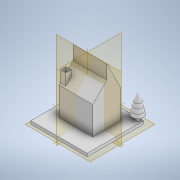
# Autodesk Inventor part: House_Assembly_Depth_Tracking
Saved by Autodesk Inventor 2022.4 (Build 264492010, 492A)
## iProperties
Created: 2025-04-13
Part Number: House_Assembly_Depth_Tracking
Material: Generic
Document SubType Name: Modeling
Designer: jan-m
Density: 1 g/cm^3
Appearance: Default
Author: jan-m
Autodesk Inventor part; units mm, degrees
sketch "Sketch1" plane through (0, 0, 0) normal (1, 0, 0) x (0, 1, 0)
  line L0 (11, 100) -> (0, 100)
  line L1 (0, 100) -> (0, -100)
  line L2 (0, -100) -> (11, -100)
  line L3 (11, -100) -> (11, 100)
  line L4 (-2.2, 0) -> (13.2, 0) projected
  line L5 (0, 140) -> (0, -140) projected
  point P0 (0, 0)
  point P1 (11, 0)
  dimension "d0" = 200
  dimension "d1" = 11
  dimension "d2" = 0
  constraints: 8 end point, 2 parallel, 1 horizontal, 1 midpoint, 1 perpendicular, 1 point on line
  measures "d0" distance of L2.end L0.start
  measures "d1" distance of L1.end L2.end
  measures "d2" distance between parallel lines of L5 L1
extrude "Extrusion1" add sketch "Sketch1" along normal mid plane 200
sketch "Sketch2" plane through (0, 0, 0) normal (1, 0, 0) x (0, 1, 0)
  line L0 (111, 40) -> (11, 40)
  line L1 (11, 40) -> (11, -60)
  line L2 (11, -60) -> (111, -60)
  line L3 (111, -60) -> (111, 40)
  line L4 (-32.1032, 0) -> (192.619, 0) projected
  line L5 (11, -100) -> (11, 100) projected
  line L6 (111, 40) -> (161, 40)
  line L7 (161, 40) -> (161, -10)
  line L8 (161, -10) -> (111, -10)
  line L9 (111, -10) -> (111, 40)
  line L10 (111, -60) -> (211, -60)
  line L11 (211, -60) -> (211, -10)
  line L12 (211, -10) -> (111, -10)
  line L13 (111, -10) -> (111, -60)
  line L14 (111, 40) -> (161, -10)
  line L15 (111, -60) -> (211, -10)
  point P0 (0, 0)
  dimension "d5" = 100
  dimension "d6" = 40
  dimension "d7" = 100
  dimension "d8" = 0
  dimension "d9" = 50
  dimension "d10" = 50
  dimension "d11" = 100
  dimension "d12" = 50
  constraints: 28 end point, 6 parallel, 3 horizontal, 3 perpendicular
  measures "d5" distance of L1.end L2.end
  measures "d6" distance between parallel lines of L4 L0
  measures "d7" distance of L2.end L0.start
  measures "d8" distance between parallel lines of L5 L1
  measures "d9" distance of L7.end L8.end
  measures "d10" distance of L6.end L7.end
  measures "d11" distance of L12.end L11.end
  measures "d12" distance of L11.end L10.end
extrude "Extrusion2" add sketch "Sketch2" along normal mid plane 120 contours L3 L4 L1 L0 | L14 L4 L3 | L4 L14 L8 L3 | L3 L2 L1 L4 | L8 L12 L15 L3
sketch "Sketch3" plane through (-60, 0, 0) normal (-1, 0, 0) x (0, 0, 1)
  line L0 (15.607, 155.393) -> (35.607, 155.393)
  line L1 (35.607, 155.393) -> (35.607, 135.393)
  line L2 (35.607, 135.393) -> (15.607, 135.393)
  line L3 (15.607, 135.393) -> (15.607, 155.393)
  line L4 (40, 111) -> (-10, 161) projected
  line L5 (35.607, 135.393) -> (35.607, 115.393)
  line L6 (-10, 161) -> (40, 111) projected
  line L7 (15.607, 135.393) -> (35.607, 115.393)
  point P0 (0, 0)
  dimension "d15" = 20
  dimension "d16" = 20
  dimension "d17" = 4.393
  constraints: 12 end point, 2 parallel, 2 point on line, 1 horizontal, 1 perpendicular, 1 vertical
  measures "d15" distance of L1.end L2.end
  measures "d16" distance of L0.end L1.end
  measures "d17" distance from line of L4.start L5
extrude "Extrusion3" add sketch "Sketch3" against normal blind 20
sketch "Sketch4" plane through (-60, 155.393, 35.607) normal (0, 1, 0) x (1, 0, 0)
  line L0 (20, 20) -> (20, 0) projected
  line L1 (0, 20) -> (20, 20) projected
  line L2 (0, 0) -> (0, 20) projected
  line L3 (0, 0) -> (20, 0) projected
  line L4 (18, 2) -> (18, 18)
  line L5 (18, 18) -> (2, 18)
  line L6 (2, 18) -> (2, 2)
  line L7 (2, 2) -> (18, 2)
  point P0 (60, 35.607)
  dimension "d20" = 2
  constraints: 8 end point, 3 other
  measures "d20" distance between parallel lines of L0 L4
extrude "Extrusion4" cut sketch "Sketch4" against normal blind 20 contours L7 L6 L5 L4
sketch "Sketch5" plane through (-100, 11, 100) normal (0, 1, 0) x (1, 0, 0)
  line L0 (200, 200) -> (200, 0) projected
  line L1 (0, 200) -> (200, 200) projected
  point P0 (100, 100)
  point P1 (190, 190)
  dimension "d23" = 10
  dimension "d24" = 10
  measures "d23" distance from line of L0 point (190, 190)
  measures "d24" distance from line of L1 point (190, 190)
ref_plane "Work Plane1" through (90, 11, -90) normal (1, 0, 0) x (0, 1, 0)
sketch "Sketch7" plane through (90, 11, -90) normal (1, 0, 0) x (0, 1, 0)
  line L0 (0, -10) -> (0, 190) projected
  line L1 (0, 0) -> (20, 0)
  line L2 (20, 0) -> (20, 5)
  line L3 (20, 5) -> (0, 5)
  line L4 (0, 5) -> (0, 0)
  line L5 (20, 0) -> (20, 20)
  line L6 (90, 0) -> (60.481, 11.7284)
  line L7 (60.481, 11.7284) -> (60.481, 5)
  line L8 (60.481, 9.4368) -> (46.541, 14.9754)
  line L9 (46.541, 14.9754) -> (46.541, 5)
  line L10 (46.541, 12.5046) -> (32.601, 18.0432)
  line L11 (32.601, 18.0432) -> (32.601, 5)
  line L12 (32.601, 15.2739) -> (20, 20)
  line L13 (90, 0) -> (20, 0)
  point P0 (-11, 90)
  dimension "d25" = 20
  dimension "d26" = 5
  dimension "d27" = 20
  dimension "d28" = 15
  dimension "d29" = 15
  constraints: 26 end point, 4 parallel, 3 point on line, 2 horizontal, 1 perpendicular, 1 vertical
  measures "d25" distance of L3.end L2.end
  measures "d26" distance of L2.end L1.end
  measures "d27" distance of L1.end L5.end
  measures "d28" distance of L8.start L8.end
  measures "d29" distance of L10.start L10.end
revolve "Revolution1" add sketch "Sketch7" angle 360 about axis through (90, 101, -90) along (0, -1, 0)
body "Solid1"
